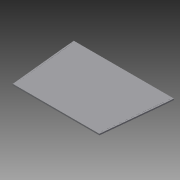
# Autodesk Inventor part: Char Support Base
Saved by Autodesk Inventor 2015 (Build 190159000, 159)
## iProperties
Created: 2016-03-22
Part Number: Char Support Base
Material: Generic
Document SubType Name: Modeling
Designer: Mac
Density: 1 g/cm^3
Appearance: Default
Author: Mac
Autodesk Inventor part; units mm, degrees
ref_plane "YZ Plane" through (0, 0, 0) normal (1, 0, 0) x (0, 1, 0)
ref_plane "XZ Plane" through (0, 0, 0) normal (0, 1, 0) x (-1, 0, 0)
ref_plane "XY Plane" through (0, 0, 0) normal (0, 0, 1) x (1, 0, 0)
sketch "Sketch1" plane through (0, 0, 0) normal (0, 1, 0) x (-1, 0, 0)
  line L0 (227.7416, -361.3719) -> (255.6062, -89.335) projected
  line L1 (255.6062, -89.335) -> (666.7545, -89.335) projected
  line L2 (666.7545, -89.335) -> (694.6192, -361.372) projected
  line L3 (694.6192, -361.372) -> (698.5066, -407.7253) projected
  line L4 (223.8542, -407.7253) -> (698.5066, -407.7253) projected
  line L5 (227.7416, -361.3719) -> (223.8542, -407.7253) projected
  line L6 (428.6458, -367.8211) -> (493.715, -367.8211) projected
  arc A0 (493.715, -367.8211) -> (493.715, -354.9226) centre (493.715, -361.3719) ccw projected
  line L7 (493.715, -354.9226) -> (428.6458, -354.9226) projected
  arc A1 (428.6458, -354.9226) -> (428.6458, -367.8211) centre (428.6458, -361.3719) ccw projected
  line L8 (666.7545, -89.335) -> (698.5066, -407.7253)
  line L9 (223.8542, -407.7253) -> (255.6062, -89.335)
  line L10 (705.4115, -414.0753) -> (700.9421, -360.7831)
  line L11 (700.9421, -360.7831) -> (672.4873, -82.985)
  line L12 (672.4873, -82.985) -> (249.8734, -82.985)
  line L13 (249.8734, -82.985) -> (221.4187, -360.7829)
  line L14 (221.4187, -360.7829) -> (216.9493, -414.0753)
  line L15 (216.9493, -414.0753) -> (705.4115, -414.0753)
  point P0 (0, 0)
  dimension "d0" = 6.35
  constraints: 16 end point, 5 other
  measures "d0" distance between parallel lines of L15 L4
extrude "Extrusion1" add sketch "Sketch1" along normal blind 6.35 contours L1 L8 L4 L9 | A1 L7 A0 L6 | L15 L14 L13 L12 L11 L10
body "Solid1"
